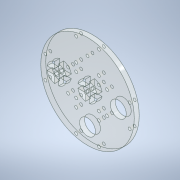
# Autodesk Inventor part: Bottom_Plate_For_Valve
Saved by Autodesk Inventor 2020 (Build 240168000, 168)
## iProperties
Created: 2021-06-26
Part Number: Bottom_Plate_For_Valve
Material: Glass
Document SubType Name: Modeling
Designer: Workshop
Density: 2.18 g/cm^3
Appearance: Clear
Author: Workshop
Autodesk Inventor part; units mm, degrees
ref_plane "YZ Plane" through (0, 0, 0) normal (1, 0, 0) x (0, 1, 0)
ref_plane "XZ Plane" through (0, 0, 0) normal (0, 1, 0) x (-1, 0, 0)
ref_plane "XY Plane" through (0, 0, 0) normal (0, 0, 1) x (1, 0, 0)
sketch "Sketch1" plane through (0, 0, 0) normal (0, 0, 1) x (1, 0, 0)
  circle A0 centre (19.5736, 11.4021) radius 1.5 projected
  line L0 (2.052, 3.5186) -> (2.052, 9.6538) projected
  arc A1 (9.6607, 2.019) -> (2.052, 9.6538) centre (0, 0) ccw projected
  line L1 (9.6607, 2.019) -> (3.5411, 2.0129) projected
  arc A2 (3.5411, 2.0129) -> (2.052, 3.5186) centre (0, 0) ccw projected
  circle A3 centre (11.4021, 11.4021) radius 1.5 projected
  circle A4 centre (11.4021, 19.5737) radius 1.5 projected
  circle A5 centre (42.3778, 11.4021) radius 1.5 projected
  line L2 (2.052, -3.5186) -> (2.052, -9.6538) projected
  arc A6 (2.052, -9.6538) -> (9.6607, -2.019) centre (0, 0) ccw projected
  line L3 (9.6607, -2.019) -> (3.5411, -2.0129) projected
  arc A7 (2.052, -3.5186) -> (3.5411, -2.0129) centre (0, 0) ccw projected
  circle A8 centre (0, -30.9758) radius 8 projected
  circle A9 centre (30.9758, 0) radius 8 projected
  circle A10 centre (42.3779, -11.4021) radius 1.5 projected
  circle A11 centre (19.5737, -11.4021) radius 1.5 projected
  circle A12 centre (0, 0) radius 1.5 projected
  line L4 (-2.052, 3.5186) -> (-2.052, 9.6538) projected
  arc A13 (-2.052, 9.6538) -> (-9.6607, 2.019) centre (0, 0) ccw projected
  line L5 (-9.6607, 2.019) -> (-3.5411, 2.0129) projected
  arc A14 (-2.052, 3.5186) -> (-3.5411, 2.0129) centre (0, 0) ccw projected
  line L6 (-2.052, -3.5186) -> (-2.052, -9.6538) projected
  arc A15 (-9.6607, -2.019) -> (-2.052, -9.6538) centre (0, 0) ccw projected
  line L7 (-9.6607, -2.019) -> (-3.5411, -2.0129) projected
  arc A16 (-3.5411, -2.0129) -> (-2.052, -3.5186) centre (0, 0) ccw projected
  circle A17 centre (11.4021, -19.5736) radius 1.5 projected
  circle A18 centre (-11.4021, 19.5736) radius 1.5 projected
  circle A19 centre (-11.4021, 11.4021) radius 1.5 projected
  circle A20 centre (0, 0) radius 47 projected
  circle A21 centre (11.4021, -42.3778) radius 1.5 projected
  circle A22 centre (-11.4021, -11.4021) radius 1.5 projected
  circle A23 centre (-11.4021, -19.5737) radius 1.5 projected
  circle A24 centre (-11.4021, -42.3779) radius 1.5 projected
  circle A25 centre (-19.5736, -11.4021) radius 1.5 projected
  line L8 (-28.9238, -3.5186) -> (-28.9238, -9.6538) projected
  arc A26 (-28.9238, -9.6538) -> (-21.3151, -2.019) centre (-30.9758, 0) ccw projected
  line L9 (-21.3151, -2.019) -> (-27.4347, -2.0129) projected
  arc A27 (-28.9238, -3.5186) -> (-27.4347, -2.0129) centre (-30.9758, 0) ccw projected
  line L10 (-33.0277, -3.5186) -> (-33.0277, -9.6538) projected
  arc A28 (-40.6365, -2.019) -> (-33.0277, -9.6538) centre (-30.9758, 0) ccw projected
  line L11 (-40.6365, -2.019) -> (-34.5169, -2.0129) projected
  arc A29 (-34.5169, -2.0129) -> (-33.0277, -3.5186) centre (-30.9758, 0) ccw projected
  circle A30 centre (-42.3778, -11.4021) radius 1.5 projected
  circle A31 centre (-19.5737, 11.4021) radius 1.5 projected
  circle A32 centre (11.4021, -11.4021) radius 1.5 projected
  circle A33 centre (-42.3779, 11.4021) radius 1.5 projected
  circle A34 centre (-11.4021, 42.3778) radius 1.5 projected
  circle A35 centre (0, 30.9758) radius 1.5 projected
  circle A36 centre (11.4021, 42.3779) radius 1.5 projected
  line L12 (-28.9238, 3.5186) -> (-28.9238, 9.6538) projected
  arc A37 (-21.3151, 2.019) -> (-28.9238, 9.6538) centre (-30.9758, 0) ccw projected
  line L13 (-21.3151, 2.019) -> (-27.4347, 2.0129) projected
  arc A38 (-27.4347, 2.0129) -> (-28.9238, 3.5186) centre (-30.9758, 0) ccw projected
  circle A39 centre (-30.9758, 0) radius 2.25 projected
  line L14 (-33.0277, 3.5186) -> (-33.0277, 9.6538) projected
  arc A40 (-33.0277, 9.6538) -> (-40.6365, 2.019) centre (-30.9758, 0) ccw projected
  line L15 (-40.6365, 2.019) -> (-34.5169, 2.0129) projected
  arc A41 (-33.0277, 3.5186) -> (-34.5169, 2.0129) centre (-30.9758, 0) ccw projected
extrude "Extrusion1" add sketch "Sketch1" along normal mid plane 5
body "Solid1"
